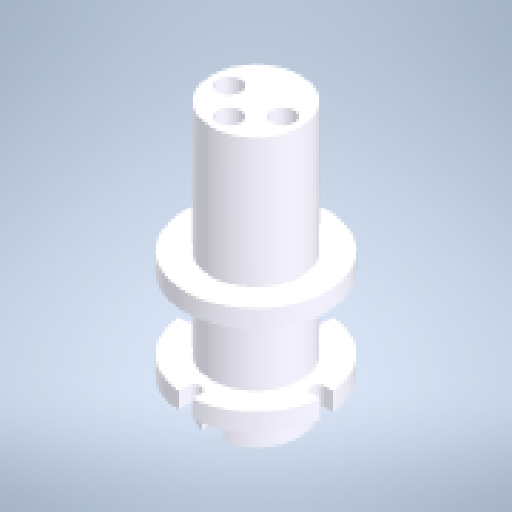
# Autodesk Inventor part: 033
Saved by Autodesk Inventor 2023 (Build 270158000, 158)
## iProperties
Created: 2022-04-13
Part Number: 033
Material: Glass
Document SubType Name: Modeling
Designer: Vinicius Miguel
Density: 2.18 g/cm^3
Appearance: Cool White
Author: Vinicius Miguel
Autodesk Inventor part; units mm, degrees
ref_plane "YZ Plane" through (0, 0, 0) normal (1, 0, 0) x (0, 1, 0)
ref_plane "XZ Plane" through (0, 0, 0) normal (0, 1, 0) x (-1, 0, 0)
ref_plane "XY Plane" through (0, 0, 0) normal (0, 0, 1) x (1, 0, 0)
sketch "Sketch5" plane through (0, 0, 0) normal (0, 0, 1) x (1, 0, 0)
  line L0 (0, 0) -> (0, 60)
  line L1 (0, 0) -> (10, 0)
  line L2 (10, 0) -> (10, 7)
  line L3 (10, 7) -> (15.85, 7)
  line L4 (15.85, 7) -> (15.85, 11)
  line L5 (15.85, 11) -> (10, 11)
  line L6 (10, 11) -> (10, 27)
  line L7 (10, 27) -> (15.85, 27)
  line L8 (15.85, 31) -> (10, 31)
  line L9 (10, 31) -> (10, 60)
  line L10 (10, 60) -> (0, 60)
  line L11 (15.85, 31) -> (15.85, 27)
  dimension "d17" = 31.7
  dimension "d18" = 7
  dimension "d19" = 4
  dimension "d23" = 20
  dimension "d26" = 60
  dimension "d27" = 20
  dimension "d48" = 31.7
  dimension "d49" = 16
  dimension "d50" = 4
  constraints: 24 end point, 8 perpendicular, 2 vertical, 2 vertical alignment, 1 horizontal
  measures "d17" diameter of L4 L0
  measures "d18" distance of L1.end L2.end
  measures "d19" distance of L3.end L4.end
  measures "d23" diameter of L6 L0
  measures "d26" distance of L0.start L0.end
  measures "d27" diameter of L2 L0
  measures "d48" diameter of L11 L0
  measures "d49" distance of L5.end L6.end
  measures "d50" distance of L8.start L7.end
revolve "Revolution1" add sketch "Sketch5" angle 360 about axis through (0, 0, 0) along (0, 1, 0)
sketch "Sketch6" plane through (0, 0, 0) normal (0, -1, 0) x (1, 0, 0)
  line L0 (-6, 0) -> (6, 0)
  circle A0 centre (0, 6) radius 4
  point P0 (0, 0)
  point P1 (6, 0)
  point P2 (0, 0)
  dimension "d29" = 12
  dimension "d56" = 8
  dimension "d57" = 6
  constraints: 4 coincident, 2 end point, 1 centre point, 1 horizontal, 1 midpoint, 1 vertical alignment
  measures "d29" distance of L0.start L0.end
  measures "d56" diameter of A0
  measures "d57" distance of A0.centre point (0, 0)
hole "Hole2" at (6, 0, 0) at (-6, 0, 0) at (0, 0, 6) direction (0, 1, 0) diameter 3 end through all counterbore diameter 5 counterbore depth 15
sketch "Sketch8" plane through (0, 7, 0) normal (0, -1, 0) x (1, 0, 0)
  line L0 (-17.88, 0) -> (-13.88, 0) construction
  line L1 (-17.88, 1.5) -> (-13.88, 1.5)
  line L2 (-13.88, -1.5) -> (-17.88, -1.5)
  arc A0 (-17.88, 1.5) -> (-17.88, -1.5) centre (-17.88, 0) ccw
  arc A1 (-13.88, -1.5) -> (-13.88, 1.5) centre (-13.88, 0) ccw
  point P0 (0, 0)
  point P1 (-15.88, 0)
  dimension "d40" = 13.88
  dimension "d41" = 1.5
  dimension "d42" = 4
  constraints: 8 end point, 4 point on circle, 4 tangent, 2 centre point, 1 horizontal, 1 midpoint, 1 parallel
  measures "d40" distance of L0.end point (0, 0)
  measures "d41" radius of A0
  measures "d42" distance of L0.start L0.end
extrude "Extrusion5" cut sketch "Sketch8" against normal up to surface (4 mm away)
pattern_circular "Circular Pattern1" count 4 over 360 about axis through (0, 3.5, 0) along (0, 1, 0) of "Extrusion5"
sketch "Sketch9" plane through (0, 60, 0) normal (0, 1, 0) x (1, 0, 0)
  circle A0 centre (-6, 0) radius 1.5 projected
  circle A1 centre (6, 0) radius 1.5 projected
  circle A2 centre (-6, 0) radius 2.5
  circle A3 centre (6, 0) radius 1.5 projected
  circle A4 centre (6, 0) radius 2.5
  circle A5 centre (0, -6) radius 1.5 projected
  circle A6 centre (0, -6) radius 1.5 projected
  circle A7 centre (0, -6) radius 2.5
  point P0 (0, 0)
  point P1 (0, 0)
  dimension "d51" = 5
  dimension "d53" = 5
  dimension "d68" = 5
  constraints: 3 centre point, 3 coincident
  measures "d51" diameter of A2
  measures "d53" diameter of A4
  measures "d68" diameter of A7
extrude "Extrusion6" cut sketch "Sketch9" against normal blind 15 contours A2 | A4 | A5 | A7
sketch "Sketch10" plane through (0, 0, 0) normal (0, -1, 0) x (1, 0, 0)
  point P0 (0, 0)
  point P1 (0, 0)
  constraints: 1 coincident
hole "Hole3" at (0, 0, 0) direction (0, 1, 0) diameter 3 depth 10 tip angle 118
sketch "Sketch11" plane through (0, 0, 0) normal (0, -1, 0) x (1, 0, 0)
  circle A0 centre (0, 6) radius 2.5 projected
  line L0 (0, 6) -> (0, 17) construction
  line L1 (-2.5, 6) -> (-2.5, 17)
  line L2 (2.5, 17) -> (2.5, 6)
  arc A1 (-2.5, 6) -> (2.5, 6) centre (0, 6) ccw
  arc A2 (2.5, 17) -> (-2.5, 17) centre (0, 17) ccw
  point P0 (0, 0)
  point P1 (0, 11.5)
  point P2 (-2.5, 6)
  point P3 (2.5, 6)
  dimension "d65" = 11
  constraints: 8 end point, 4 point on circle, 4 tangent, 2 centre point, 1 concentric, 1 midpoint, 1 parallel, 1 vertical
  measures "d65" distance of L0.start L0.end
extrude "Extrusion7" cut sketch "Sketch11" against normal blind 7.5 contours A0 L1 A2 L2
body "Solid2"
